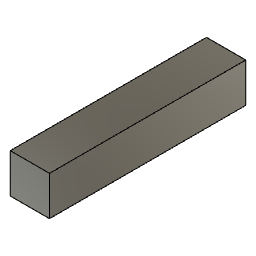
basic_piano_key (Autodesk Fusion 360 design; units mm, degrees)
Autodesk Fusion 360 part; units mm, degrees
sketch "Sketch1" plane through (0, 0, 0) normal (0, 0, 1) x (1, 0, 0)
  line L0 (0, 0) -> (25.4, 0)
  line L1 (25.4, 0) -> (25.4, 127)
  line L2 (25.4, 127) -> (0, 127)
  line L3 (0, 127) -> (0, 0)
  line L4 (1, 126) -> (24.4, 126)
  line L5 (24.4, 126) -> (24.4, 1)
  line L6 (24.4, 1) -> (1, 1)
  line L7 (1, 1) -> (1, 126)
  line L8 (2, 125) -> (23.4, 125)
  line L9 (23.4, 125) -> (23.4, 2)
  line L10 (23.4, 2) -> (2, 2)
  line L11 (2, 2) -> (2, 125)
  dimension "d1" = 25.4
  dimension "d2" = 127
  dimension "d3" = 23.4
  dimension "d4" = 125
  dimension "d5" = 1
  dimension "d6" = 1
  dimension "d7" = 21.4
  dimension "d8" = 123
  dimension "d9" = 1
  dimension "d10" = 1
  constraint horizontal L0
  constraint vertical L1
  constraint horizontal L2
  constraint vertical L3
  constraint coincident L0.start L3.end
  constraint horizontal L4
  constraint vertical L5
  constraint horizontal L6
  constraint vertical L7
  constraint horizontal L8
  constraint vertical L9
  constraint horizontal L10
  constraint vertical L11
  measures "d1" distance of L0.start L0.end
  measures "d2" distance of L0.start L2.end
  measures "d3" distance of L4.start L4.end
  measures "d4" distance of L4.start L6.end
  measures "d5" distance of L2 L4
  measures "d6" distance of L3 L7
  measures "d7" distance of L8.start L8.end
  measures "d8" distance of L8.start L10.end
  measures "d9" distance of L4 L8
  measures "d10" distance of L7 L11
extrude "Extrude1" add sketch "Sketch1" along normal blind 25.4 contours L0 L1 L2 L3 | L4 L5 L6 L7 | L8 L9 L10 L11
sketch "Sketch2" plane through (0, 0, 0) normal (0, 0, -1) x (1, 0, 0)
  line L0 (0, 0) -> (0, -127)
  line L1 (0, -127) -> (25.4, -127)
  line L2 (25.4, -127) -> (25.4, 0)
  line L3 (25.4, 0) -> (0, 0)
  line L4 (24.4, -126) -> (1, -126)
  line L5 (1, -126) -> (1, -1)
  line L6 (1, -1) -> (24.4, -1)
  line L7 (24.4, -1) -> (24.4, -126)
  line L8 (23.4, -125) -> (2, -125)
  line L9 (2, -125) -> (2, -2)
  line L10 (2, -2) -> (23.4, -2)
  line L11 (23.4, -2) -> (23.4, -125)
  dimension "d13" = 23.4
  dimension "d14" = 125
  dimension "d15" = 1
  dimension "d16" = 1
  dimension "d17" = 21.4
  dimension "d18" = 123
  dimension "d19" = 1
  dimension "d20" = 1
  constraint horizontal L4
  constraint vertical L5
  constraint horizontal L6
  constraint vertical L7
  constraint horizontal L8
  constraint vertical L9
  constraint horizontal L10
  constraint vertical L11
  measures "d13" distance of L4.start L4.end
  measures "d14" distance of L4.start L6.end
  measures "d15" distance of L1 L4
  measures "d16" distance of L2 L7
  measures "d17" distance of L8.start L8.end
  measures "d18" distance of L8.start L10.end
  measures "d19" distance of L4 L8
  measures "d20" distance of L7 L11
extrude "Extrude2" cut sketch "Sketch2" against normal blind 24.4 draft -0.5 contours L4 L5 L6 L7
extrude "Extrude3" cut 1 faces at (16.2667, 43, 0) along direction (0, 0, 1) blind 13
delete_face "DeleteFace1" 1 faces at (2, 84, 4.3333)
delete_face "DeleteFace2" 1 faces at (9.0955, 125, 8.6667)
delete_face "DeleteFace3" 1 faces at (23.4, 84.0378, 8.6667)
delete_face "DeleteFace4" 1 faces at (16.2667, 2, 8.6667)
